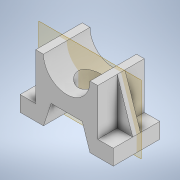
# Autodesk Inventor part: ПЧ2021
Saved by Autodesk Inventor 2021.1 (Build 251245010, 245A)
## iProperties
Created: 2023-10-25
Part Number: ПЧ2021
Material: Типовые
Document SubType Name: Modeling
Designer: Lenovo
Density: 1 g/cm^3
Appearance: По умолчанию
Author: Lenovo
Autodesk Inventor part; units mm, degrees
ref_plane "YZ Plane" through (0, 0, 0) normal (1, 0, 0) x (0, 1, 0)
ref_plane "XZ Plane" through (0, 0, 0) normal (0, 1, 0) x (-1, 0, 0)
sketch "Эскиз1" plane through (0, 0, 0) normal (0, 0, 1) x (1, 0, 0)
  line L0 (-60, 0) -> (-60, 20)
  line L1 (-60, 20) -> (-40, 20)
  line L2 (-40, 20) -> (-40, 80)
  line L3 (-40, 80) -> (-30, 80)
  line L4 (-30, 0) -> (-20, 30)
  line L5 (-20, 30) -> (20, 30)
  line L6 (30, 0) -> (20, 30)
  line L7 (-60, 0) -> (-30, 0)
  line L8 (60, 0) -> (60, 20)
  line L9 (60, 20) -> (40, 20)
  line L10 (40, 20) -> (40, 80)
  line L11 (40, 80) -> (30, 80)
  line L12 (30, 0) -> (20, 30)
  line L13 (20, 30) -> (-20, 30)
  line L14 (60, 0) -> (30, 0)
  arc A0 (-30, 80) -> (30, 80) centre (0, 80) ccw
  point P0 (0, 0)
  constraints: 30 end point, 3 perpendicular, 2 horizontal, 2 point on circle, 1 centre point
extrude "Выдавливание1" add sketch "Эскиз1" against normal blind 60
sketch "Эскиз3" plane through (0, 0, 0) normal (0, 1, 0) x (-1, 0, 0)
  line L0 (-20, -60) -> (20, -60) projected
  circle A0 centre (0, -30) radius 15
  point P0 (0, 0)
  dimension "d16" = 30
  constraints: 1 centre point
  measures "d16" diameter of A0
extrude "Выдавливание2" cut sketch "Эскиз3" along normal mid plane 1000
ref_plane "РабПлоскость1" through (0, 0, -30) normal (0, 0, 1) x (1, 0, 0)
sketch "Эскиз4" plane through (0, 0, -30) normal (0, 0, 1) x (1, 0, 0)
  line L0 (60, 0) -> (60, 20) projected
  line L1 (40, 80) -> (30, 80) projected
  line L2 (0, 0) -> (0, 80)
  line L3 (-60, 20) -> (-40, 80)
  line L4 (-60, 0) -> (-60, 20) projected
  line L5 (-60, 20) -> (-40, 20)
  line L6 (-40, 20) -> (-40, 80) projected
  line L7 (-40, 20) -> (-40, 80)
  line L8 (60, 20) -> (40, 80)
  line L9 (60, 20) -> (40, 20)
  line L10 (40, 20) -> (40, 80)
  constraints: 14 end point, 3 symmetric about line, 1 horizontal, 1 perpendicular, 1 vertical
extrude "Выдавливание3" add sketch "Эскиз4" along normal mid plane 10
